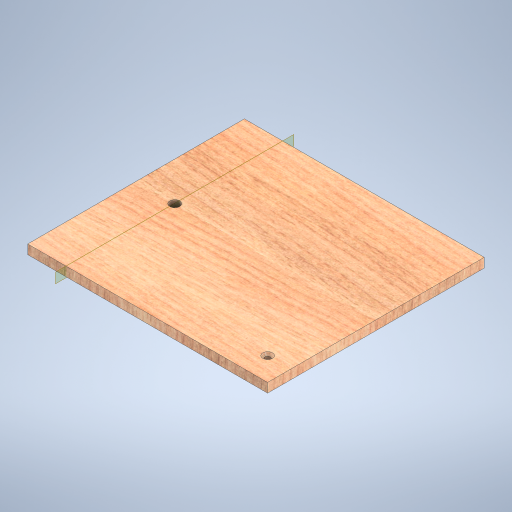
# Autodesk Inventor part: base_plates
Saved by Autodesk Inventor 2024.1 (Build 281209000, 209)
## iProperties
Created: 2022-10-18
Part Number: base_plates
Material: Wood (Birch)
Document SubType Name: Modeling
Designer: 박동준
Density: 0.55 g/cm^3
Appearance: Birch - Natural Polished
Sheet Metal Rule: Default_mm
Author: 박동준
Autodesk Inventor part; units mm, degrees
ref_plane "YZ Plane" through (0, 0, 0) normal (1, 0, 0) x (0, 1, 0)
ref_plane "XZ Plane" through (0, 0, 0) normal (0, 1, 0) x (-1, 0, 0)
ref_plane "XY Plane" through (0, 0, 0) normal (0, 0, 1) x (1, 0, 0)
sketch "스케치1" plane through (0, 0, 0) normal (0, 1, 0) x (-1, 0, 0)
  line L0 (125, -140) -> (-125, -140)
  line L1 (-125, -140) -> (-125, 140)
  line L2 (-125, 140) -> (125, 140)
  line L3 (125, 140) -> (125, -140)
  point P0 (0, 0)
  point P1 (125, 0)
  point P2 (0, -140)
  dimension "d0" = 250
  dimension "d1" = 280
  constraints: 8 end point, 2 midpoint, 2 parallel, 1 horizontal, 1 horizontal alignment, 1 perpendicular, 1 vertical alignment
  measures "d0" distance of L1.end L2.end
  measures "d1" distance of L0.end L1.end
extrude "돌출1" add sketch "스케치1" along normal mid plane 12
sketch "Sketch3" plane through (0, 6, 0) normal (0, 1, 0) x (1, 0, 0)
  line L0 (-125, 140) -> (-125, -140) projected
  line L1 (-125, 140) -> (-185, 140)
  line L2 (-185, 140) -> (-185, -140)
  line L3 (-185, -140) -> (-125, -140)
  line L4 (-125, -140) -> (-125, 140)
  point P0 (0, 0)
  point P1 (-125, -140)
  dimension "d7" = 60
  dimension "d8" = 280
  constraints: 8 end point, 2 parallel, 1 horizontal, 1 perpendicular
  measures "d7" distance of L3.end L2.end
  measures "d8" distance of L2.end L1.end
extrude "Extrusion2" add sketch "Sketch3" against normal up to surface (12 mm away)
sketch "Sketch5" plane through (0, 6, 0) normal (0, 1, 0) x (1, 0, 0)
  circle A0 centre (-135, 0) radius 6.4
  point P0 (0, 0)
  constraints: 1 centre point, 2 other
extrude "Extrusion3" cut sketch "Sketch5" against normal blind 10
sketch "Sketch6" plane through (0, 6, 0) normal (0, 1, 0) x (1, 0, 0)
  circle A0 centre (-135, 0) radius 6.4 projected
  line L0 (-185, -140) -> (125, -140) projected
  line L1 (125, -140) -> (125, 140) projected
  line L2 (125, 140) -> (-185, 140) projected
  line L3 (-185, 140) -> (-185, -140) projected
  point P0 (0, 0)
  point P1 (95, -110)
  dimension "d20" = 30
  dimension "d21" = 30
  measures "d20" distance from line of L1 point (95, -110)
  measures "d21" distance from line of L0 point (95, -110)
hole "Hole2" at (95, 6, 110) direction (0, -1, 0) diameter 6.6 end through all countersink diameter 12.6 countersink angle 90 clearance for "Countersunk Flat Head Screw ISO 2009/7046" size "M6" standard "ISO"
ref_plane "Work Plane1" through (-135, 6, -140) normal (-1, 0, 0) x (0, 0, 1)
equation "\"TransitionRadius\" = BendRadius"
equation "\"BendRadius\" = 0.5"
